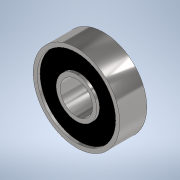
# Autodesk Inventor part: 6201 Bearing
Saved by Autodesk Inventor 2022 (Build 260153000, 153)
## iProperties
Created: 2022-08-17
Part Number: 6201 Bearing
Material: Generic
Document SubType Name: Modeling
Designer: Nick
Density: 1 g/cm^3
Appearance: Steel - Polished
Author: Nick
Autodesk Inventor part; units mm, degrees
ref_plane "YZ Plane" through (0, 0, 0) normal (1, 0, 0) x (0, 1, 0)
ref_plane "XZ Plane" through (0, 0, 0) normal (0, 1, 0) x (-1, 0, 0)
sketch "Sketch1" plane through (0, 0, 0) normal (0, 0, 1) x (1, 0, 0)
  circle A0 centre (0, 0) radius 6
  circle A1 centre (0, 0) radius 16
  dimension "d0" = 12
  dimension "d1" = 32
  constraints: 2 centre point, 2 coincident
  measures "d0" diameter of A0
  measures "d1" diameter of A1
extrude "Extrusion1" add sketch "Sketch1" along normal blind 10
sketch "Sketch2" plane through (0, 0, 10) normal (0, 0, 1) x (1, 0, 0)
  circle A0 centre (0, 0) radius 16 projected
  circle A1 centre (0, 0) radius 6 projected
  circle A2 centre (0, 0) radius 7.5
  circle A3 centre (0, 0) radius 14.5
  dimension "d4" = 1.5
  dimension "d5" = 1.5
  constraints: 2 centre point
  measures "d4" radial gap between concentric circles of A1 A2
  measures "d5" radial gap between concentric circles of A0 A3
extrude "Extrusion2" cut sketch "Sketch2" against normal blind 1 contours A3
ref_plane "Work Plane1" through (0, 0, 5) normal (0, 0, 1) x (1, 0, 0)
mirror "Mirror1" about plane through (0, 0, 5) normal (0, 0, 1) of "Extrusion2"
body "Solid1"
